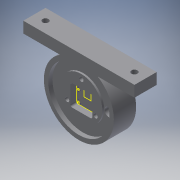
# Autodesk Inventor part: basicMount
Saved by Autodesk Inventor 2019.3 (Build 233278000, 278)
## iProperties
Created: 2019-01-13
Part Number: basicMount
Material: Generic
Document SubType Name: Modeling
Designer: steele
Density: 1 g/cm^3
Appearance: Default
Author: steele
Autodesk Inventor part; units mm, degrees
ref_plane "YZ Plane" through (0, 0, 0) normal (1, 0, 0) x (0, 1, 0)
ref_plane "XZ Plane" through (0, 0, 0) normal (0, 1, 0) x (-1, 0, 0)
ref_plane "XY Plane" through (0, 0, 0) normal (0, 0, 1) x (1, 0, 0)
sketch "Sketch1" plane through (0, 0, 0) normal (0, 0, 1) x (1, 0, 0)
  line L0 (63.5, -6.35) -> (63.5, 6.35)
  line L1 (63.5, 6.35) -> (-63.5, 6.35)
  line L2 (-63.5, 6.35) -> (-63.5, -6.35)
  line L3 (0, 0) -> (0, -40) construction
  line L4 (-63.5, -6.35) -> (-21.6259, -6.35)
  line L5 (21.6259, -6.35) -> (63.5, -6.35)
  line L6 (-63.5, -6.35) -> (-6.9307, -0.6931) construction
  line L7 (0, 0) -> (63.5, 6.35) construction
  line L8 (63.5, -6.35) -> (6.9307, -0.6931) construction
  line L9 (0, 0) -> (-63.5, 6.35) construction
  arc A0 (-21.6259, -6.35) -> (21.6259, -6.35) centre (0, -40) ccw
  line L10 (63.5, 0) -> (-63.5, 0) construction
  dimension "d0" = 127
  dimension "d1" = 12.7
  dimension "d2" = 40
  dimension "d31" = 6.35
  dimension "d32" = 40
  constraints: 22 end point, 3 parallel, 2 horizontal, 2 midpoint, 2 perpendicular, 2 point on circle, 1 centre point, 1 coincident, 1 point on line, 1 vertical
  measures "d0" distance of L2.end L0.start
  measures "d1" distance of L0.end L0.start
  measures "d2" distance of L3.start L3.end
  measures "d31" distance from line of L1 L3.start
  measures "d32" radius of A0
extrude "Extrusion1" add sketch "Sketch1" against normal blind 25.4
sketch "Sketch2" plane through (0, 0, 0) normal (0, 0, 1) x (1, 0, 0)
  arc A0 (-21.6259, -6.35) -> (21.6259, -6.35) centre (0, -40) ccw projected
  circle A1 centre (0, -40) radius 35
  point P0 (0, 0)
  dimension "d6" = 70
  constraints: 1 centre point, 1 coincident
  measures "d6" diameter of A1
extrude "Extrusion2" cut sketch "Sketch2" against normal blind 2.794
sketch "Sketch3" plane through (0, -40, -2.794) normal (0, 0, 1) x (1, 0, 0)
  circle A0 centre (0, 0) radius 35 projected
  circle A1 centre (0, 0) radius 31
  circle A2 centre (0, 0) radius 24
  point P0 (0, 40)
  dimension "d9" = 62
  dimension "d10" = 48
  constraints: 2 centre point, 2 coincident
  measures "d9" diameter of A1
  measures "d10" diameter of A2
extrude "Extrusion3" cut sketch "Sketch3" against normal blind 2 contours A0 | A1
sketch "Sketch4" plane through (0, -40, -4.794) normal (0, 0, 1) x (1, 0, 0)
  circle A0 centre (0, 0) radius 35 construction
  line L0 (0, 0) -> (34.925, 0) construction
  circle A1 centre (29.5, 0) radius 5
  point P0 (0, 40)
  dimension "d33" = 29.5
  dimension "d34" = 10
  constraints: 2 end point, 1 centre point, 1 horizontal, 1 point on line
  measures "d33" distance of A1.centre L0.start
  measures "d34" diameter of A1
extrude "Extrusion4" cut sketch "Sketch4" against normal through all
sketch "Sketch5" plane through (-63.5, -6.35, 0) normal (0, -1, 0) x (1, 0, 0)
  line L0 (0, 0) -> (0, -25.4) construction
  line L1 (0, -12.7) -> (127, -12.7) construction
  line L2 (127, 0) -> (127, -25.4) construction
  point P0 (63.5, 0)
  point P1 (12.7, -12.7)
  point P2 (114.3, -12.7)
  dimension "d15" = 12.7
  dimension "d16" = 12.7
  constraints: 2 end point, 2 midpoint, 2 point on line
  measures "d15" distance from line of point (12.7, -12.7) L0
  measures "d16" distance from line of point (114.3, -12.7) L2
hole "Hole1" at (-50.8, -6.35, -12.7) at (50.8, -6.35, -12.7) direction (0, 1, 0) diameter 6.7564 end through all counterbore diameter 8.0264 counterbore depth 9.525 clearance for "Hex Head Bolt" size "1/4" standard "Ansi Unified Screw Threads"
sketch "Sketch6" plane through (0, 0, -25.4) normal (0, 0, -1) x (-1, 0, 0)
  circle A0 centre (-29.5, -40) radius 5 projected
  line L0 (63.5, -6.35) -> (63.5, 6.35) projected
  line L1 (63.5, 6.35) -> (-63.5, 6.35) projected
  line L2 (-63.5, 6.35) -> (-63.5, -6.35) projected
  line L3 (-63.5, -6.35) -> (-21.6259, -6.35) projected
  arc A1 (-21.6259, -6.35) -> (21.6259, -6.35) centre (0, -40) ccw projected
  line L4 (21.6259, -6.35) -> (63.5, -6.35) projected
  line L5 (1.1662, -29.21) -> (1.1662, -40.2844) projected
  line L6 (3.1474, -29.21) -> (1.1662, -29.21) projected
  line L7 (3.1474, -40.2844) -> (3.1474, -29.21) projected
  line L8 (3.1474, -40.2844) -> (16.4443, -40.2844) projected
  line L9 (16.4443, -40.2844) -> (16.4443, 3.9878) projected
  arc A2 (16.4443, 3.9878) -> (14.0821, 6.35) centre (14.0821, 3.9878) ccw projected
  line L10 (-9.7685, 6.35) -> (14.0821, 6.35) projected
  arc A3 (-9.7685, 6.35) -> (-12.1307, 3.9878) centre (-9.7685, 3.9878) ccw projected
  line L11 (-12.1307, -40.2844) -> (-12.1307, 3.9878) projected
  line L12 (-12.1307, -40.2844) -> (1.1662, -40.2844) projected
  line L13 (13.4998, -8.7122) -> (13.4998, -24.5872) projected
  line L14 (13.4998, -24.5872) -> (-9.1862, -24.5872) projected
  line L15 (-9.1862, -24.5872) -> (-9.1862, -8.7122) projected
  line L16 (-9.1862, -8.7122) -> (13.4998, -8.7122) projected
  circle A4 centre (-8.9557, 0.8128) radius 1.6256 projected
  circle A5 centre (13.2693, -34.1122) radius 1.6256 projected
  circle A6 centre (13.2693, 0.8128) radius 1.6256 projected
  circle A7 centre (-8.9557, -34.1122) radius 1.6256 projected
  point P0 (0, 0)
  constraints: 4 coincident
hole "Hole2" at (-13.2693, 0.8128, -25.4) at (-13.2693, -34.1122, -25.4) at (8.9557, -34.1122, -25.4) at (8.9557, 0.8128, -25.4) direction (0, 0, 1) diameter 3.5052 depth 12.7 tip angle 118 counterbore diameter 4.8514 counterbore depth 7.1374
sketch "Sketch8" plane through (0, -40, -2.794) normal (0, 0, 1) x (1, 0, 0)
  circle A0 centre (-16.2398, -9.376) radius 1.905 projected
  circle A1 centre (0, 18.7521) radius 1.905 projected
  circle A2 centre (16.2398, -9.3761) radius 1.905 projected
  line L0 (22.8154, -16.5062) -> (18.8007, -20.9651) projected
  line L1 (18.8007, -20.9651) -> (15.8281, -18.2886) projected
  line L2 (15.8281, -18.2886) -> (19.8429, -13.8297) projected
  line L3 (19.8429, -13.8297) -> (22.8154, -16.5062) projected
  line L4 (27.533, 5.9104) -> (28.1602, -0.0568) projected
  line L5 (28.1602, -0.0568) -> (24.1821, -0.4749) projected
  line L6 (24.1821, -0.4749) -> (23.5549, 5.4922) projected
  line L7 (23.5549, 5.4922) -> (27.533, 5.9104) projected
  line L8 (14.0309, 24.4158) -> (18.885, 20.8891) projected
  line L9 (18.885, 20.8891) -> (16.5339, 17.6531) projected
  line L10 (16.5339, 17.6531) -> (11.6798, 21.1798) projected
  line L11 (11.6798, 21.1798) -> (14.0309, 24.4158) projected
  line L12 (-8.756, 26.7644) -> (-2.8871, 28.0119) projected
  line L13 (-2.8871, 28.0119) -> (-2.0554, 24.0993) projected
  line L14 (-2.0554, 24.0993) -> (-7.9243, 22.8518) projected
  line L15 (-7.9243, 22.8518) -> (-8.756, 26.7644) projected
  line L16 (-25.7487, 11.4019) -> (-22.7487, 16.5981) projected
  line L17 (-22.7487, 16.5981) -> (-19.2846, 14.5981) projected
  line L18 (-19.2846, 14.5981) -> (-22.2846, 9.4019) projected
  line L19 (-22.2846, 9.4019) -> (-25.7487, 11.4019) projected
  line L20 (-25.7025, -11.5056) -> (-27.5566, -5.7993) projected
  line L21 (-27.5566, -5.7993) -> (-23.7524, -4.5632) projected
  line L22 (-23.7524, -4.5632) -> (-21.8983, -10.2696) projected
  line L23 (-21.8983, -10.2696) -> (-25.7025, -11.5056) projected
  line L24 (-8.648, -26.7995) -> (-14.1293, -24.3591) projected
  line L25 (-14.1293, -24.3591) -> (-12.5023, -20.7049) projected
  line L26 (-12.5023, -20.7049) -> (-7.021, -23.1453) projected
  line L27 (-7.021, -23.1453) -> (-8.648, -26.7995) projected
  line L28 (3, -24) -> (3, -28) projected
  line L29 (3, -28) -> (-3, -28) projected
  line L30 (-3, -28) -> (-3, -24) projected
  line L31 (-3, -24) -> (3, -24) projected
  line L32 (-18.8007, -20.9651) -> (-22.8154, -16.5062) projected
  line L33 (-22.8154, -16.5062) -> (-19.8429, -13.8297) projected
  line L34 (-19.8429, -13.8297) -> (-15.8281, -18.2886) projected
  line L35 (-15.8281, -18.2886) -> (-18.8007, -20.9651) projected
  line L36 (-28.1602, -0.0568) -> (-27.533, 5.9104) projected
  line L37 (-27.533, 5.9104) -> (-23.5549, 5.4922) projected
  line L38 (-23.5549, 5.4922) -> (-24.1821, -0.4749) projected
  line L39 (-24.1821, -0.4749) -> (-28.1602, -0.0568) projected
  line L40 (-18.885, 20.8891) -> (-14.0309, 24.4158) projected
  line L41 (-14.0309, 24.4158) -> (-11.6798, 21.1798) projected
  line L42 (-11.6798, 21.1798) -> (-16.5339, 17.6531) projected
  line L43 (-16.5339, 17.6531) -> (-18.885, 20.8891) projected
  line L44 (2.8871, 28.0119) -> (8.756, 26.7644) projected
  line L45 (8.756, 26.7644) -> (7.9243, 22.8518) projected
  line L46 (7.9243, 22.8518) -> (2.0554, 24.0993) projected
  line L47 (2.0554, 24.0993) -> (2.8871, 28.0119) projected
  line L48 (22.7487, 16.5981) -> (25.7487, 11.4019) projected
  line L49 (25.7487, 11.4019) -> (22.2846, 9.4019) projected
  line L50 (22.2846, 9.4019) -> (19.2846, 14.5981) projected
  line L51 (19.2846, 14.5981) -> (22.7487, 16.5981) projected
  line L52 (27.5566, -5.7993) -> (25.7025, -11.5056) projected
  line L53 (25.7025, -11.5056) -> (21.8983, -10.2696) projected
  line L54 (21.8983, -10.2696) -> (23.7524, -4.5632) projected
  line L55 (23.7524, -4.5632) -> (27.5566, -5.7993) projected
  line L56 (14.1293, -24.3591) -> (8.648, -26.7995) projected
  line L57 (8.648, -26.7995) -> (7.021, -23.1453) projected
  line L58 (7.021, -23.1453) -> (12.5023, -20.7049) projected
  line L59 (12.5023, -20.7049) -> (14.1293, -24.3591) projected
  line L60 (5, 5) -> (5, -5) projected
  line L61 (5, -5) -> (-5, -5) projected
  line L62 (-5, -5) -> (-5, 5) projected
  line L63 (-5, 5) -> (5, 5) projected
  circle A3 centre (0, 0) radius 34 projected
  point P0 (0, 40)
  constraints: 3 coincident
hole "Hole3" at (0, -21.2479, -2.794) at (-16.2398, -49.376, -2.794) at (16.2398, -49.3761, -2.794) direction (0, 0, -1) diameter 3.5052 depth 12.7 tip angle 118 counterbore diameter 4.8514 counterbore depth 7.1374
sketch "Sketch10" plane through (0, -40, -2.794) normal (0, 0, 1) x (1, 0, 0)
  line L0 (-4, -4) -> (-4, 4) projected
  line L1 (-4, 4) -> (4, 4) projected
  line L2 (4, 4) -> (4, -4) projected
  line L3 (4, -4) -> (-4, -4) projected
  circle A0 centre (10.5, -12.5) radius 1.1 projected
  circle A1 centre (10.5, 0.08) radius 1.1 projected
  circle A2 centre (-10.5, 0.08) radius 1.1 projected
  circle A3 centre (-10.5, -12.5) radius 1.1 projected
  arc A4 (-12.5, -12.5) -> (-10.5, -14.5) centre (-10.5, -12.5) ccw projected
  line L4 (-10.5, -14.5) -> (10.5, -14.5) projected
  arc A5 (10.5, -14.5) -> (12.5, -12.5) centre (10.5, -12.5) ccw projected
  line L5 (12.5, -12.5) -> (12.5, 7.542) projected
  arc A6 (12.5, 7.542) -> (10.5, 9.542) centre (10.5, 7.542) ccw projected
  line L6 (10.5, 9.542) -> (-10.5, 9.542) projected
  arc A7 (-10.5, 9.542) -> (-12.5, 7.542) centre (-10.5, 7.542) ccw projected
  line L7 (-12.5, 7.542) -> (-12.5, -12.5) projected
  line L8 (-13.5, 10.542) -> (13.5, 10.542)
  circle A8 centre (0, 0) radius 24 projected
  line L9 (-13.5, -15.5) -> (-13.5, 10.542)
  line L10 (-13.5, -15.5) -> (13.5, -15.5)
  line L11 (13.5, 10.542) -> (13.5, -15.5)
  point P0 (0, 40)
  dimension "d54" = 1
  dimension "d55" = 1
  dimension "d56" = 1
  dimension "d57" = 1
  constraints: 8 end point, 2 parallel, 1 horizontal, 1 perpendicular
  measures "d54" distance between parallel lines of L8 L6
  measures "d55" distance between parallel lines of L10 L4
  measures "d56" distance between parallel lines of L7 L9
  measures "d57" distance between parallel lines of L11 L5
ref_plane "Work Plane1" through (0, -40, -9.794) normal (0, 0, 1) x (1, 0, 0)
sketch "Sketch11" plane through (0, -40, -9.794) normal (0, 0, 1) x (1, 0, 0)
  line L0 (-4, -4) -> (-4, 4) projected
  line L1 (-4, 4) -> (4, 4) projected
  line L2 (4, 4) -> (4, -4) projected
  line L3 (4, -4) -> (-4, -4) projected
  circle A0 centre (10.5, -12.5) radius 1.1 projected
  circle A1 centre (10.5, 0.08) radius 1.1 projected
  circle A2 centre (-10.5, 0.08) radius 1.1 projected
  circle A3 centre (-10.5, -12.5) radius 1.1 projected
  arc A4 (-12.5, -12.5) -> (-10.5, -14.5) centre (-10.5, -12.5) ccw projected
  line L4 (-10.5, -14.5) -> (10.5, -14.5) projected
  arc A5 (10.5, -14.5) -> (12.5, -12.5) centre (10.5, -12.5) ccw projected
  line L5 (12.5, -12.5) -> (12.5, 7.542) projected
  arc A6 (12.5, 7.542) -> (10.5, 9.542) centre (10.5, 7.542) ccw projected
  line L6 (10.5, 9.542) -> (-10.5, 9.542) projected
  arc A7 (-10.5, 9.542) -> (-12.5, 7.542) centre (-10.5, 7.542) ccw projected
  line L7 (-12.5, 7.542) -> (-12.5, -12.5) projected
  point P0 (0, 40)
  constraints: 4 coincident
hole "Hole4" at (-10.5, -39.92, -9.794) at (10.5, -39.92, -9.794) at (10.5, -52.5, -9.794) at (-10.5, -52.5, -9.794) direction (0, 0, -1) diameter 3.5052 depth 12.7 tip angle 118 counterbore diameter 4.8514 counterbore depth 7.1374
extrude "Extrusion7" cut sketch "Sketch10" against normal blind 7 contours L0 L1 L2 L3 | A0 | A1 | A2 | A3 | L7 A7 L6 A6 L5 A5 L4 A4 | L8 L11 L10 L9
body "Solid1"
